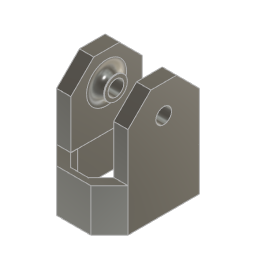
idler bracket (Autodesk Fusion 360 design; units mm, degrees)
Autodesk Fusion 360 part; units mm, degrees
note: some values were not read from the file. Chosen so that the rebuilt part matches the saved one: which bodies a step acts on.
sketch "Sketch1" plane through (0, 0, 0) normal (0, 0, 1) x (1, 0, 0)
  line L0 (12.5, -12.5) -> (-12.5, -12.5)
  line L1 (-12.5, -12.5) -> (-12.5, 12.5)
  line L2 (-12.5, 12.5) -> (12.5, 12.5)
  line L3 (12.5, 12.5) -> (12.5, -12.5)
  line L4 (12.5, -12.5) -> (-12.5, 12.5) construction
  line L5 (-12.5, -12.5) -> (12.5, 12.5) construction
  line L6 (10.05, -10.05) -> (-10.05, -10.05)
  line L7 (-10.05, -10.05) -> (-10.05, 10.05)
  line L8 (-10.05, 10.05) -> (10.05, 10.05)
  line L9 (10.05, 10.05) -> (10.05, -10.05)
  line L10 (10.05, -10.05) -> (-10.05, 10.05) construction
  line L11 (-10.05, -10.05) -> (10.05, 10.05) construction
  dimension "d3" = 25
  dimension "d4" = 25
  dimension "d5" = 20.1
  dimension "d6" = 20.1
  constraint horizontal L0
  constraint perpendicular L0 L1
  constraint parallel L0 L2
  constraint parallel L1 L3
  constraint coincident L4 origin
  constraint coincident L5 origin
  constraint horizontal L6
  constraint perpendicular L6 L7
  constraint parallel L6 L8
  constraint parallel L7 L9
  constraint coincident L10 origin
  constraint coincident L11 origin
  measures "d3" distance of L1.end L2.end
  measures "d4" distance of L0.end L1.end
  measures "d5" distance of L7.end L8.end
  measures "d6" distance of L6.end L7.end
extrude "Extrude1" add sketch "Sketch1" along normal blind 15 makes body 1
sketch "Sketch2" plane through (0, 0, 15) normal (0, 0, 1) x (-1, 0, 0)
  line L0 (10.05, -10.05) -> (-10.05, -10.05)
  line L1 (-10.05, -10.05) -> (-10.05, 10.05)
  line L2 (-10.05, 10.05) -> (10.05, 10.05)
  line L3 (10.05, 10.05) -> (10.05, -10.05)
  line L4 (-12.5, -12.5) -> (12.5, -12.5)
  line L5 (12.5, -12.5) -> (12.5, 12.5)
  line L6 (12.5, 12.5) -> (-12.5, 12.5)
  line L7 (-12.5, 12.5) -> (-12.5, -12.5)
  line L8 (12.5, -12.5) -> (7.5, -12.5)
  line L9 (7.5, -12.5) -> (7.5, 12.5)
  line L10 (7.5, 12.5) -> (12.5, 12.5)
  line L11 (12.5, 12.5) -> (12.5, -12.5)
  line L12 (-12.5, -12.5) -> (-7.5, -12.5)
  line L13 (-7.5, -12.5) -> (-7.5, 12.5)
  line L14 (-7.5, 12.5) -> (-12.5, 12.5)
  line L15 (-12.5, 12.5) -> (-12.5, -12.5)
  dimension "d9" = 5
  dimension "d10" = 5
  constraint horizontal L8
  constraint vertical L9
  constraint horizontal L10
  constraint vertical L11
  constraint coincident L4.end L5.start
  constraint horizontal L12
  constraint vertical L13
  constraint horizontal L14
  constraint vertical L15
  constraint coincident L4.start L7.end
  measures "d9" distance of L4.end L8.end
  measures "d10" distance of L4.start L12.end
extrude "Extrude2" add sketch "Sketch2" along normal blind 25 contours L0 L2 L3 L4 L5 L6 L8 L9 L10 L11 | L0 L2 L3 L9 | L0 L1 L2 L4 L6 L7 L12 L13 L14 L15 | L0 L1 L2 L13 bodies 1
sketch "Sketch3" plane through (-12.5, 0, 0) normal (-1, 0, 0) x (0, -1, 0)
  line L0 (-12.5, 0) -> (12.5, 0)
  line L1 (12.5, 0) -> (12.5, 40)
  line L2 (12.5, 40) -> (-12.5, 40)
  line L3 (-12.5, 40) -> (-12.5, 0)
  line L4 (0, 40) -> (0, 0) construction
  line L5 (4, 32.3094) -> (0, 34.6188)
  line L6 (0, 34.6188) -> (-4, 32.3094)
  line L7 (-4, 32.3094) -> (-4, 27.6906)
  line L8 (-4, 27.6906) -> (0, 25.3812)
  line L9 (0, 25.3812) -> (4, 27.6906)
  line L10 (4, 27.6906) -> (4, 32.3094)
  point P0 (0, 30)
  point P1 (0, 30)
  dimension "d13" = 10
  dimension "d27" = 4
  constraint midpoint L2 L4.start
  constraint coincident L4.end origin
  constraint coincident L4 P1
  constraint coincident P1 P0
  constraint vertical L10
  measures "d13" distance of L4.start P1
  measures "d27" distance of P1 L10
hole "Hole1" at (-12.5, 0, 30) direction (1, 0, 0) diameter 5.5 end through all bodies 1
sketch "Sketch4" plane through (-7.5, 0, 0) normal (1, 0, 0) x (0, 1, 0)
  circle A0 centre (0, 30) radius 2.75
  line L0 (10.05, 15) -> (12.5, 15)
  line L1 (12.5, 15) -> (12.5, 40)
  line L2 (12.5, 40) -> (-12.5, 40)
  line L3 (-12.5, 40) -> (-12.5, 15)
  line L4 (-12.5, 15) -> (-10.05, 15)
  line L5 (-10.05, 15) -> (10.05, 15)
  circle A1 centre (0, 30) radius 4
  dimension "d17" = 8
  constraint concentric A0 A1
  measures "d17" diameter of A1
sketch "Sketch5" plane through (7.5, 0, 0) normal (-1, 0, 0) x (0, -1, 0)
  circle A0 centre (0, 30) radius 2.75
  line L0 (-12.5, 15) -> (-10.05, 15)
  line L1 (-10.05, 15) -> (10.05, 15)
  line L2 (10.05, 15) -> (12.5, 15)
  line L3 (12.5, 15) -> (12.5, 40)
  line L4 (12.5, 40) -> (-12.5, 40)
  line L5 (-12.5, 40) -> (-12.5, 15)
  circle A1 centre (0, 30) radius 4
  dimension "d22" = 8
  constraint concentric A0 A1
  measures "d22" diameter of A1
extrude "Extrude3" add sketch "Sketch4" along normal blind 3.275 contours A1 bodies 1
extrude "Extrude4" add sketch "Sketch5" along normal blind 3.275 contours A1 bodies 1
fillet "Fillet2" radius 3 2 edges at (7.5, 3.7293, 31.4465) (-7.5, -3.7293, 31.4465) on bodies 1
extrude "Extrude5" cut sketch "Sketch3" against normal blind 3.5 contours L5 L6 L7 L8 L9 L10 bodies 1
sketch "Sketch6" plane through (0, 0, 0) normal (0, 0, -1) x (1, 0, 0)
  line L0 (10.05, -10.05) -> (-10.05, -10.05)
  line L1 (-10.05, -10.05) -> (-10.05, 10.05)
  line L2 (-10.05, 10.05) -> (10.05, 10.05)
  line L3 (10.05, 10.05) -> (10.05, -10.05)
  line L4 (-12.5, -12.5) -> (12.5, -12.5)
  line L5 (12.5, -12.5) -> (12.5, 12.5)
  line L6 (12.5, 12.5) -> (-12.5, 12.5)
  line L7 (-12.5, 12.5) -> (-12.5, -12.5)
  line L8 (-7.5, -10.05) -> (-7.5, 10.05)
  line L9 (7.5, -10.05) -> (7.5, 10.05)
  line L10 (-12.5, 12.5) -> (-6, 19)
  line L11 (-6, 19) -> (0, 19)
  line L12 (0, 19) -> (0, 17)
  line L13 (-10.05, 10.05) -> (-3.1, 17)
  line L14 (0, 17) -> (-3.1, 17)
  line L15 (-7.6, 10.05) -> (-7.6, 12.5)
  line L16 (0, -1.75) -> (0, -22.5)
  line L17 (0, 17) -> (3.1, 17)
  line L18 (6, 19) -> (0, 19)
  line L19 (0, 19) -> (0, 17)
  line L20 (10.05, 10.05) -> (3.1, 17)
  line L21 (12.5, 12.5) -> (6, 19)
  line L22 (7.6, 10.05) -> (7.6, 12.5)
  line L23 (1.75, 0) -> (22.5, 0)
  line L24 (10.05, -10.05) -> (3.1, -17)
  line L25 (7.6, -10.05) -> (7.6, -12.5)
  line L26 (12.5, -12.5) -> (6, -19)
  line L27 (6, -19) -> (0, -19)
  line L28 (0, -17) -> (3.1, -17)
  line L29 (0, -17) -> (-3.1, -17)
  line L30 (-6, -19) -> (0, -19)
  line L31 (-12.5, -12.5) -> (-6, -19)
  line L32 (-10.05, -10.05) -> (-3.1, -17)
  line L33 (-7.6, -10.05) -> (-7.6, -12.5)
  dimension "d30" = 2
  dimension "d31" = 45
  dimension "d37" = 6.5
  constraint coincident L6.end L7.start
  constraint perpendicular L7 L11
  constraint perpendicular L11 L12
  constraint coincident L1.end L2.start
  constraint horizontal L14
  constraint parallel L10 L13
  constraint coincident L13 L15.end
  constraint coincident L6 L15.end
  constraint coincident L2 L15.start
  constraint vertical L15
  constraint symmetric L6.end L16 L5.end
  constraint symmetric L10.end L16 L18.start
  constraint symmetric L11.end L16 L12.start
  constraint symmetric L12.end L16 L14.start
  constraint symmetric L1.end L16 L2.end
  constraint symmetric L13.end L16 L17.end
  constraint symmetric L15.start L16 L22.start
  constraint symmetric L15.end L16 L22.end
  constraint symmetric L6.end L23 L4.start
  constraint symmetric L10.end L23 L30.start
  constraint symmetric L11.end L23 L27.end
  constraint symmetric L12.end L23 L28.start
  constraint symmetric L1.end L23 L0.end
  constraint symmetric L13.end L23 L29.end
  constraint symmetric L15.start L23 L33.start
  constraint symmetric L15.end L23 L33.end
  constraint symmetric L17.end L23 L24.end
  constraint symmetric L18.start L23 L26.end
  constraint symmetric L2.end L23 L0.start
  constraint symmetric L5.end L23 L4.end
  constraint symmetric L22.start L23 L25.start
  constraint symmetric L22.end L23 L25.end
  measures "d30" distance of L11.end L12.end
  measures "d31" angle of L6 L13
  measures "d37" distance of L6.end L11
extrude "Extrude6" cut sketch "Sketch6" against normal blind 15 contours L0 L4 L16 L25 | L0 L4 L16 L33 | L2 L6 L15 L22 bodies 1 makes body 2 at (12.5, 0, 9.0833)
extrude "Extrude7" add sketch "Sketch6" against normal blind 15 contours L4 L16 L24 L26 L27 L28 | L6 L12 L17 L18 L19 L20 L21 | L4 L16 L29 L30 L31 L32 | L6 L10 L11 L12 L13 L14 L19 bodies 1 2
chamfer "Chamfer1" distance 8 angle 45 4 edges at (10, -12.5, 40) (-10, -12.5, 40) (-10, 12.5, 40) (10, 12.5, 40) on bodies 1 2
fillet "Fillet1" [suppressed]
